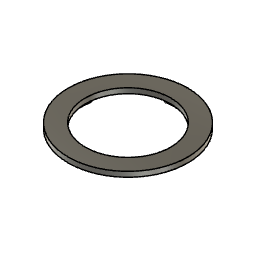
lampshade_holder (Autodesk Fusion 360 design; units mm, degrees)
Autodesk Fusion 360 part; units mm, degrees
sketch "Sketch1" plane through (0, 0, 0) normal (0, 0, 1) x (1, 0, 0)
  circle A0 centre (0, 0) radius 35
  circle A1 centre (0, 0) radius 25
  circle A2 centre (0, 0) radius 28 construction
  circle A3 centre (0, 0) radius 32 construction
  dimension "d1" = 70
  dimension "d2" = 50
  dimension "d6" = 56
  dimension "d15" = 4
  constraint coincident A0.centre A1.centre
  constraint concentric A0 A1
  constraint concentric A0 A2
  measures "d1" diameter of A0
  measures "d2" diameter of A1
  measures "d6" diameter of A2
extrude "Extrude1" add sketch "Sketch1" along normal blind 3
sketch "Sketch2" plane through (0, 0, 0) normal (0, 0, -1) x (1, 0, 0)
  circle A0 centre (0, 0) radius 25
  circle A1 centre (0, 0) radius 35
  circle A2 centre (0, 0) radius 28 construction
  arc A3 (4.8393, 26.6644) -> (-4.8393, 26.6644) centre (0, 0) ccw
  arc A4 (4.8393, 26.6644) -> (5.1607, 28.4355) centre (5, 27.55) ccw
  arc A5 (5.1607, 28.4355) -> (-5.1607, 28.4355) centre (0, 0) ccw
  arc A6 (-5.1607, 28.4355) -> (-4.8393, 26.6644) centre (-5, 27.55) ccw
  arc A7 (5, 27.55) -> (-5, 27.55) centre (0, 0) ccw construction
  line L0 (-5, 27.55) -> (5, 27.55) construction
  line L1 (0, 0) -> (0, 55.0999) construction
  dimension "d5" = 56
  dimension "d7" = 0.9
  dimension "d14" = 10
  constraint concentric A0 A2
  constraint tangent A3 A4
  constraint tangent A4 A5
  constraint tangent A5 A6
  constraint tangent A3 A6
  constraint coincident A0.centre A1.centre
  constraint coincident A2 A4.centre
  constraint coincident A6.centre A7.end
  constraint coincident A4.centre A7.start
  constraint vertical L1
  constraint midpoint L0 L1
  measures "d5" diameter of A2
  measures "d7" radius of A4
  measures "d14" horizontal distance of A6.centre A4.centre
extrude "Extrude2" add sketch "Sketch2" along normal blind 2.5 contours A3 A4 A5 A6
pattern_circular "C-Pattern1" count 4 over 360 about axis through (0, 0, 0) along (0, 0, -1) of "Extrude2"
